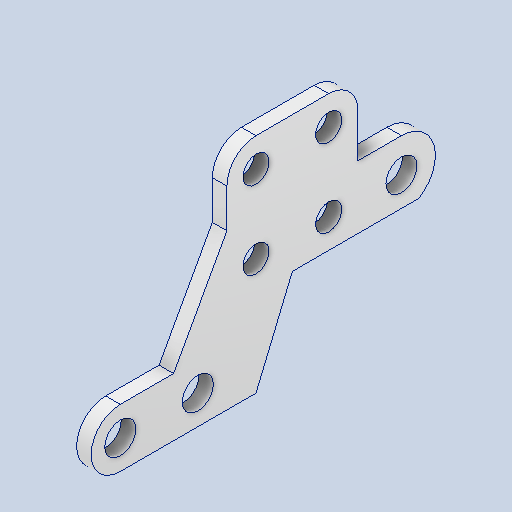
# Autodesk Inventor part: fork_outside
Saved by Autodesk Inventor 2024.1 (Build 281209000, 209)
## iProperties
Created: 2025-01-18
Part Number: fork_outside
Material: アルミニウム 6061
Document SubType Name: Sheet Metal
Designer: hibik
Density: 2.7 g/cm^3
Sheet Metal Rule: Default_mm
Appearance: アルミニウム - フラット
Author: hibik
Autodesk Inventor part; units mm, degrees
ref_plane "YZ Plane" through (0, 0, 0) normal (1, 0, 0) x (0, 1, 0)
ref_plane "XZ Plane" through (0, 0, 0) normal (0, 1, 0) x (-1, 0, 0)
ref_plane "XY Plane" through (0, 0, 0) normal (0, 0, 1) x (1, 0, 0)
sketch "スケッチ1" plane through (0, 0, 0) normal (1, 0, 0) x (0, 1, 0)
  line L0 (7, 0) -> (-7, 0)
  line L1 (-7, 0) -> (-7, -6.75)
  line L2 (-7, -6.75) -> (7, -6.75)
  line L3 (7, -6.75) -> (7, 0)
  circle A0 centre (4, -3.75) radius 3
  circle A1 centre (-4, -3.75) radius 3
  line L4 (7, -0.75) -> (-7, -0.75)
  line L5 (-7, 0) -> (-7, 6.75)
  line L6 (-7, 6.75) -> (7, 6.75)
  line L7 (7, 6.75) -> (7, 0)
  circle A2 centre (4, 3.75) radius 3
  circle A3 centre (-4, 3.75) radius 3
  line L8 (7, 0.75) -> (-7, 0.75)
  circle A4 centre (4, -3.75) radius 1.35
  circle A5 centre (-4, -3.75) radius 1.35
  circle A6 centre (-4, 3.75) radius 1.35
  circle A7 centre (4, 3.75) radius 1.35
  line L9 (0, -21.85) -> (0, 27.85)
  line L10 (-10, 20.75) -> (-16, 20.75)
  line L11 (-16, 20.75) -> (-16, 3.75)
  line L12 (-16, 3.75) -> (-10, 3.75)
  line L13 (-10, 3.75) -> (-10, 20.75)
  circle A8 centre (-13, 17.75) radius 1.6
  circle A9 centre (-13, 9.75) radius 1.6
  circle A10 centre (-13, 17.75) radius 3
  line L14 (-7, -6.75) -> (-0.5, -6.75)
  line L15 (-0.5, -6.75) -> (-0.5, -14.75)
  line L16 (-0.5, -14.75) -> (-7, -14.75)
  line L17 (-7, -14.75) -> (-7, -6.75)
  circle A11 centre (-4, -11.25) radius 1.6
  circle A12 centre (-4, -11.25) radius 3.5
  line L18 (-16, 3.75) -> (-7, 0)
  line L19 (0, 6.75) -> (-10, 12.25)
  point P0 (0, 0)
  point P1 (0, 0)
  point P2 (-4.1535, 3.75)
  point P3 (7, -3.75)
  point P4 (7, 3.75)
  point P5 (-7, 3.75)
  point P6 (-7, -3.75)
  point P7 (4, 6.75)
  point P8 (-4, 6.75)
  point P9 (-16, 17.75)
  point P10 (-7, 6.75)
  point P11 (-5.3457, 6.75)
  point P12 (-10, 17.75)
  point P13 (2.4272, 6.3046)
  point P14 (-7, 3.75)
  point P15 (-7, -13.0528)
  point P16 (-0.5, -11.25)
  point P17 (4, -6.75)
  dimension "d0" = 14
  dimension "d1" = 6
  dimension "d2" = 6
  dimension "d3" = 0.75
  dimension "d5" = 2.7
  dimension "d12" = 6
  dimension "d13" = 3.2
  dimension "d14" = 3.2
  dimension "d15" = 3
  dimension "d16" = 8
  dimension "d17" = 3
  dimension "d19" = 3.2
  dimension "d20" = 8
  dimension "d21" = 3.5
  dimension "d22" = 3
  measures "d0" distance of L1.end L2.end
  measures "d1" diameter of A0
  measures "d2" diameter of A1
  measures "d3" distance between parallel lines of L0 L4
  measures "d5" diameter of A4
  measures "d12" distance of L10.start L10.end
  measures "d13" diameter of A8
  measures "d14" diameter of A9
  measures "d15" distance from line of L6 A9.centre
  measures "d16" distance of A8.centre A9.centre
  measures "d17" distance from line of L10 A8.centre
  measures "d19" diameter of A11
  measures "d20" distance between parallel lines of L2 L16
  measures "d21" distance from line of L16 A11.centre
  measures "d22" distance between parallel lines of L5 L13
extrude "プレート1" add sketch "スケッチ1" along normal blind 1.5 contours L3 L4 L9 L0 | L0 L9 L8 L7 | L9 L4 L1 L0 | L0 L5 L8 L9 | L3 A0 L4 | L8 A2 L7 | L18 L12 L13 L19 L6 L5 | L9 L2 A1 L4 | L4 A0 L2 L9 | L9 L6 A2 L8 | L8 A3 L6 L9 | A0 | A2 | L4 A1 L1 | L5 A3 L8 | L11 A10 L13 L12 | A1 | A3 | A1 L2 L1 | L5 L6 A3 | A10 | L15 A12 L17 L2 | A12 L17 picked at (-6.5333, -11.25)
equation "\"d17\" = 0.5 * d10"
equation "\"d6\" = Thickness"
equation "\"BendRadius\" = Thickness"
equation "\"BendReliefWidth\" = Thickness"
equation "\"BendReliefDepth\" = 0.5 * Thickness"
equation "\"CornerReliefSize\" = 4 * Thickness"
equation "\"MinimumRemnant\" = 2 * Thickness"
equation "\"TransitionRadius\" = BendRadius"
equation "\"JacobiRadiusSize\" = BendRadius"
equation "\"GapSize\" = Thickness"
equation "\"d10\" = 6"
equation "\"Thickness\" = 1.5"
